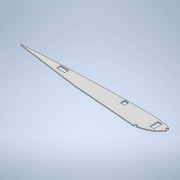
# Autodesk Inventor part: airfoil
Saved by Autodesk Inventor 2021 (Build 250183000, 183)
## iProperties
Created: 2021-03-06
Part Number: airfoil
Material: Generic
Document SubType Name: Modeling
Designer: Ferdinand Hubbard
Density: 1 g/cm^3
Appearance: Default
Author: Ferdinand Hubbard
Autodesk Inventor part; units mm, degrees
ref_plane "YZ Plane" through (0, 0, 0) normal (1, 0, 0) x (0, 1, 0)
ref_plane "XZ Plane" through (0, 0, 0) normal (0, 1, 0) x (-1, 0, 0)
ref_plane "XY Plane" through (0, 0, 0) normal (0, 0, 1) x (1, 0, 0)
sketch "Sketch1" plane through (0, 0, 0) normal (0, 1, 0) x (-1, 0, 0)
  spline S0 degree 5 poles (51.979, 34.2431) (50.8625, 34.028) (47.6122, 33.3669) (42.4356, 32.1484) (35.6445, 30.1748) (27.6551, 26.8948) (19.9185, 23.282) (13.2966, 18.4115) (8.2164, 15.1418) (4.1239, 9.095) (1.8688, 7.6936) (0.0614, 1.3934) (-0.0327, 0.731) (0.0012, -0.8157) (0.1601, -1.4322) (0.3844, -2.0614) (0.8781, -2.5552) (1.4257, -3.0265) (3.0955, -4.0074) (3.6639, -4.2019) (12.8054, -7.5819) (15.4761, -7.0321) (27.2625, -9.6881) (35.794, -9.6188) (49.4051, -10.751) (62.7459, -10.7975) (78.537, -11.1277) (95.0547, -11.0417) (112.8972, -10.9363) (131.4585, -10.6401) (150.706, -10.2647) (170.3212, -9.7779) (190.1154, -9.2196) (209.8264, -8.5865) (229.2522, -7.9015) (248.1108, -7.1621) (266.2978, -6.3832) (283.3653, -5.5497) (299.6157, -4.6319) (313.9444, -3.6518) (328.0305, -2.6976) (338.3237, -1.8152) (350.4289, -1.1113) (355.0714, -0.5725) (365.0696, -0.2501) (365.4645, -0.0704) (369.2011, -0.021) (369.9991, -0.0065) (370, 0) (370.0001, 0.0004) (369.9988, 0.0007) (369.9962, 0.0011) (369.9924, 0.0014) (369.9872, 0.0018) knots 0.394181 0.394181 0.394181 0.394181 0.394181 0.394181 0.402168 0.417605 0.432338 0.446343 0.459583 0.472 0.483512 0.493356 0.501621 0.508282 0.513504 0.517523 0.521304 0.525161 0.529372 0.535087 0.54267 0.552364 0.564195 0.578324 0.593841 0.610553 0.628313 0.64698 0.666409 0.686456 0.706982 0.727856 0.748948 0.770129 0.791274 0.812253 0.83294 0.853208 0.872937 0.892004 0.91028 0.927618 0.943841 0.958715 0.971915 0.982888 0.99083 1 1 1 1 1 1.000508 1.000508 1.000508 1.000508 1.000508 1.000508
  circle A0 centre (370, 0) radius 160 construction
  line L0 (370, 0) -> (211.4974, 21.8387)
  circle A1 centre (211.4974, 21.8387) radius 160 construction
  line L1 (211.4974, 21.8387) -> (51.979, 34.2431)
  circle A2 centre (112.1091, 11.6385) radius 9.25 construction
  line L2 (19.3886, 16.3045) -> (29.3886, 16.3045)
  line L3 (29.3886, 16.3045) -> (29.3886, -3.6955)
  line L4 (29.3886, -3.6955) -> (19.3886, -3.6955)
  line L5 (19.3886, -3.6955) -> (19.3886, 16.3045)
  line L6 (250.7844, 6.67) -> (270.7844, 6.67)
  line L7 (270.7844, 6.67) -> (270.7844, -3.33)
  line L8 (270.7844, -3.33) -> (250.7844, -3.33)
  line L9 (250.7844, -3.33) -> (250.7844, 6.67)
  line L10 (-0.096, 2.719) -> (4.904, 2.719)
  line L11 (4.904, 2.719) -> (4.904, -2.281)
  line L12 (4.904, -2.281) -> (-0.096, -2.281)
  line L13 (-0.096, -2.281) -> (-0.096, 2.719)
  circle A3 centre (369.9872, 0.0018) radius 3 construction
  line L14 (365.7713, 2.7478) -> (370.7713, 2.7478)
  line L15 (370.7713, 2.7478) -> (370.7713, -2.2522)
  line L16 (370.7713, -2.2522) -> (365.7713, -2.2522)
  line L17 (365.7713, -2.2522) -> (365.7713, 2.7478)
  line L18 (211.4974, 21.8387) -> (210.0997, -8.5616) construction
  arc A4 (200.5004, -8.8773) -> (198.939, 22.8152) centre (193.0135, 6.6385) ccw
  arc A5 (220.3414, 20.6201) -> (219.1363, -8.2496) centre (229.7182, 5.7687) ccw
  line L19 (224.7182, 10.7687) -> (234.7182, 10.7687)
  line L20 (234.7182, 10.7687) -> (234.7182, 0.7687)
  line L21 (234.7182, 0.7687) -> (224.7182, 0.7687)
  line L22 (224.7182, 0.7687) -> (224.7182, 10.7687)
  line L23 (224.7182, 10.7687) -> (234.7182, 0.7687) construction
  line L24 (234.7182, 10.7687) -> (224.7182, 0.7687) construction
  circle A6 centre (229.7182, 5.7687) radius 7.5
  line L25 (46.4065, 34.5291) -> (51.4065, 34.5291)
  line L26 (51.4065, 34.5291) -> (51.4065, 29.5291)
  line L27 (51.4065, 29.5291) -> (46.4065, 29.5291)
  line L28 (46.4065, 29.5291) -> (46.4065, 34.5291)
  line L29 (46.4065, 34.5291) -> (51.4065, 29.5291) construction
  line L30 (51.4065, 34.5291) -> (46.4065, 29.5291) construction
  circle A7 centre (229.7182, 5.7687) radius 11.5
  circle A8 centre (229.7182, 5.7687) radius 12.5
  line L31 (106.5666, 2.4214) -> (116.5666, 2.4214)
  line L32 (116.5666, 2.4214) -> (116.5666, -7.5786)
  line L33 (116.5666, -7.5786) -> (106.5666, -7.5786)
  line L34 (106.5666, -7.5786) -> (106.5666, 2.4214)
  line L35 (106.5666, 2.4214) -> (116.5666, -7.5786) construction
  line L36 (116.5666, 2.4214) -> (106.5666, -7.5786) construction
  line L37 (54.6091, 20.8885) -> (169.6091, 20.8885)
  line L38 (169.6091, 20.8885) -> (169.6091, 2.3885)
  line L39 (169.6091, 2.3885) -> (54.6091, 2.3885)
  line L40 (54.6091, 2.3885) -> (54.6091, 20.8885)
  line L41 (54.6091, 20.8885) -> (169.6091, 2.3885) construction
  line L42 (169.6091, 20.8885) -> (54.6091, 2.3885) construction
  point P0 (0, 0)
  point P1 (370, 0)
  point P2 (35.937, 30.0257)
  point P3 (27.0238, 26.4761)
  point P4 (19.2974, 22.4624)
  point P5 (12.8156, 18.139)
  point P6 (7.6237, 13.6489)
  point P7 (3.7499, 9.1521)
  point P8 (1.2115, 4.8535)
  point P9 (0.0668, 1.0195)
  point P10 (0.0003, -0.0638)
  point P11 (0.0755, -0.9849)
  point P12 (0.2106, -1.5356)
  point P13 (0.4302, -2.0122)
  point P14 (0.7739, -2.4345)
  point P15 (1.2488, -2.8423)
  point P16 (2.1566, -3.4383)
  point P17 (3.2773, -4.0196)
  point P18 (8.2772, -5.8071)
  point P19 (15.3669, -7.4261)
  point P20 (24.3167, -8.7706)
  point P21 (35.0526, -9.7678)
  point P22 (47.5438, -10.4262)
  point P23 (61.6814, -10.8267)
  point P24 (77.2847, -11.0213)
  point P25 (94.162, -11.0379)
  point P26 (112.1091, -10.9014)
  point P27 (130.911, -10.6315)
  point P28 (150.3435, -10.2474)
  point P29 (170.176, -9.7646)
  point P30 (190.1737, -9.1986)
  point P31 (229.7182, -7.8653)
  point P32 (248.7963, -7.1166)
  point P33 (267.1071, -6.3194)
  point P34 (284.4371, -5.4606)
  point P35 (300.619, -4.5258)
  point P36 (315.5184, -3.5432)
  point P37 (328.988, -2.5786)
  point P38 (340.8625, -1.7041)
  point P39 (350.9622, -0.9861)
  point P40 (359.0984, -0.4682)
  point P41 (365.0855, -0.1602)
  point P42 (368.7597, -0.0285)
  point P43 (370, 0)
  point P44 (0.4871, 2.719)
  point P45 (0.63, -2.281)
  point P46 (365.7713, -0.1232)
  point P47 (368.4073, 0.2194)
  point P48 (48.9065, 32.0291)
  point P49 (111.5666, -2.5786)
  point P50 (365.7713, 0.5826)
  point P51 (51.4065, 34.1316)
  point P52 (46.4065, 33.048)
  dimension "d5" = 160
  dimension "d8" = 160
  dimension "d10" = 18.5
  dimension "d11" = 10
  dimension "d12" = 20
  dimension "d13" = 20
  dimension "d14" = 10
  dimension "d17" = 5
  dimension "d18" = 5
  dimension "d25" = 6
  dimension "d26" = 5
  dimension "d27" = 5
  dimension "d30" = 17.2278
  dimension "d33" = 10
  dimension "d34" = 10
  dimension "d35" = 15
  dimension "d36" = 5
  dimension "d37" = 5
  dimension "d40" = 23
  dimension "d41" = 25
  dimension "d42" = 10
  dimension "d43" = 10
  dimension "d47" = 115
  dimension "d48" = 18.5
  dimension "d49" = 104.4854
  dimension "d50" = 368.7594
  constraints: 86 end point, 16 parallel, 8 horizontal, 8 midpoint, 8 perpendicular, 7 centre point, 5 coincident, 4 point on circle, 3 point on line, 55 other
  measures "d5" distance of L0.end L0.start
  measures "d8" distance of L0.end L1.end
  measures "d10" diameter of A2
  measures "d11" distance of L3.end L4.end
  measures "d12" distance of L2.end L3.end
  measures "d13" distance of L7.end L8.end
  measures "d14" distance of L6.end L7.end
  measures "d17" distance of L11.end L12.end
  measures "d18" distance of L10.end L11.end
  measures "d25" diameter of A3
  measures "d26" distance of L15.end L16.end
  measures "d27" distance of L14.end L15.end
  measures "d30" radius of A4
  measures "d33" distance of L20.end L21.end
  measures "d34" distance of L19.end L20.end
  measures "d35" diameter of A6
  measures "d36" distance of L26.end L27.end
  measures "d37" distance of L25.end L26.end
  measures "d40" diameter of A7
  measures "d41" diameter of A8
  measures "d42" distance of L32.end L33.end
  measures "d43" distance of L31.end L32.end
  measures "d47" distance of L38.end L39.end
  measures "d48" distance of L37.end L38.end
  measures "d49" horizontal distance of A2.centre point (7.624, 13.649)
  measures "d50" distance of point (368.76, -0.028) point (0, -0.064)
extrude "Extrusion3" add sketch "Sketch1" along normal blind 2 contours A4 L1 L0 A5 S0 | S0 L12 L11 L10 L28 L27 L26 L1 A4 | A5 L0 L17 S0 | L19 L20 L21 L22 | A6 | A7 | A8 | L34 L39 L40 L37 L38 L32 L31
body "Solid3"
